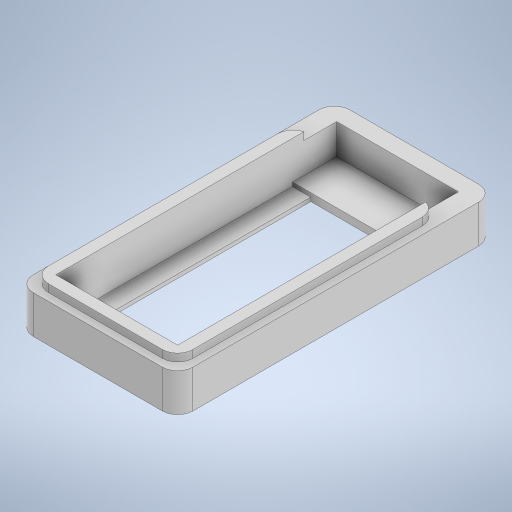
# Autodesk Inventor part: Pieza USB Tester
Saved by Autodesk Inventor 2024 (Build 280153000, 153)
## iProperties
Created: 2023-06-24
Part Number: Pieza USB Tester
Material: Genérico
Document SubType Name: Modeling
Designer: sergi
Density: 1 g/cm^3
Appearance: Valor por defecto
Author: sergi
Autodesk Inventor part; units mm, degrees
ref_plane "YZ Plane" through (0, 0, 0) normal (1, 0, 0) x (0, 1, 0)
ref_plane "XZ Plane" through (0, 0, 0) normal (0, 1, 0) x (-1, 0, 0)
ref_plane "XY Plane" through (0, 0, 0) normal (0, 0, 1) x (1, 0, 0)
sketch "Boceto1" plane through (0, 0, 0) normal (0, 1, 0) x (-1, 0, 0)
  line L0 (-8, -15.55) -> (8, -15.55)
  line L1 (8, -15.55) -> (8, 15.55)
  line L2 (8, 15.55) -> (-8, 15.55)
  line L3 (-8, 15.55) -> (-8, -15.55)
  line L4 (-8, -15.55) -> (8, 15.55) construction
  line L5 (8, -15.55) -> (-8, 15.55) construction
  line L6 (9.5, 17.05) -> (9.5, -17.05)
  line L7 (9.5, -17.05) -> (-9.5, -17.05)
  line L8 (-9.5, -17.05) -> (-9.5, 17.05)
  line L9 (-9.5, 17.05) -> (9.5, 17.05)
  point P0 (0, 0)
  dimension "d0" = 16
  dimension "d1" = 31.1
  dimension "d2" = 1.5
  constraints: 20 end point, 4 parallel, 2 midpoint, 2 perpendicular, 1 horizontal, 3 other
  measures "d0" distance of L2.end L1.end
  measures "d1" distance of L1.end L0.end
  measures "d2" distance between parallel lines of L1 L6
extrude "Extrusión1" add sketch "Boceto1" along normal blind 6
sketch "Boceto2" plane through (0, 0, 0) normal (0, -1, 0) x (1, 0, 0)
  line L0 (9.5, 17.05) -> (9.5, -17.05) projected
  line L1 (-9.5, 17.05) -> (9.5, 17.05) projected
  line L2 (-9.5, -17.05) -> (-9.5, 17.05) projected
  line L3 (9.5, -17.05) -> (-9.5, -17.05) projected
  line L4 (8, -15.55) -> (8, 15.55) projected
  line L5 (-8, -15.55) -> (8, -15.55) projected
  line L6 (-8, 15.55) -> (-8, -15.55) projected
  line L7 (8, 15.55) -> (-8, 15.55) projected
  line L8 (10.5, 18.05) -> (10.5, -18.05)
  line L9 (10.5, -18.05) -> (-10.5, -18.05)
  line L10 (-10.5, -18.05) -> (-10.5, 18.05)
  line L11 (-10.5, 18.05) -> (10.5, 18.05)
  line L12 (10.5, -18.05) -> (-10.5, -18.05)
  line L13 (-10.5, -18.05) -> (-10.5, -24.55)
  line L14 (-10.5, -24.55) -> (10.5, -24.55)
  line L15 (10.5, -24.55) -> (10.5, -18.05)
  point P0 (0, 0)
  dimension "d5" = 2.5
  dimension "d19" = 6.5
  constraints: 16 end point, 2 parallel, 1 horizontal, 1 perpendicular, 3 other
  measures "d5" distance between parallel lines of L4 L8
  measures "d19" distance of L13.end L12.end
extrude "Extrusión2" add sketch "Boceto2" against normal blind 5 contours L0 L3 L2 L1 | L8 L9 L10 L11
sketch "Boceto8" plane through (0, 0, 0) normal (0, -1, 0) x (1, 0, 0)
  line L0 (10.5, 18.05) -> (10.5, -18.05) projected
  line L1 (10.5, -18.05) -> (-10.5, -18.05)
  line L2 (-10.5, -18.05) -> (-10.5, -23.55)
  line L3 (-10.5, -23.55) -> (10.5, -23.55)
  line L4 (10.5, -23.55) -> (10.5, -18.05)
  point P0 (0, 0)
  dimension "d20" = 21
  dimension "d21" = 5.5
  constraints: 8 end point, 2 parallel, 1 horizontal, 1 perpendicular
  measures "d20" distance of L3.end L2.end
  measures "d21" distance of L2.end L1.end
extrude "Extrusión7" add sketch "Boceto8" against normal blind 5
sketch "Boceto9" plane through (0, 6, 0) normal (0, 1, 0) x (1, 0, 0)
  line L0 (9.5, -17.05) -> (9.5, 17.05) projected
  line L1 (9.5, 17.05) -> (-9.5, 17.05) projected
  line L2 (-9.5, 17.05) -> (-9.5, -17.05) projected
  line L3 (-9.5, -17.05) -> (9.5, -17.05) projected
  line L4 (8, 15.55) -> (8, -15.55) projected
  line L5 (8, -15.55) -> (-8, -15.55) projected
  line L6 (-8, -15.55) -> (-8, 15.55) projected
  line L7 (-8, 15.55) -> (8, 15.55) projected
  line L8 (-10.5, 23.55) -> (-10.5, -18.05) projected
  line L9 (-10.5, -18.05) -> (10.5, -18.05) projected
  line L10 (10.5, -18.05) -> (10.5, 23.55) projected
  line L11 (10.5, 23.55) -> (-10.5, 23.55) projected
  line L12 (-9.5, -17.05) -> (9.5, -17.05) projected
  line L13 (-9.5, 17.05) -> (-9.5, -17.05) projected
  line L14 (9.5, 17.05) -> (-9.5, 17.05) projected
  line L15 (9.5, -17.05) -> (9.5, 17.05) projected
  line L16 (-8, 15.55) -> (8, 15.55)
  line L17 (8, 15.55) -> (8, 21.35)
  line L18 (8, 21.35) -> (-8, 21.35)
  line L19 (-8, 21.35) -> (-8, 15.55)
  point P0 (0, 0)
  point P1 (8, 15.55)
  dimension "d24" = 5.8
  constraints: 8 end point, 2 parallel, 1 horizontal, 1 perpendicular
  measures "d24" distance of L17.end L16.end
extrude "Extrusión8" cut sketch "Boceto9" against normal blind 5 contours L17 L7 L19 L1 | L1 L19 L18 L17
fillet "Empalme3" radius 2 4 edges at (-10.5, 2.5, 18.05) (10.5, 2.5, 18.05) (-10.5, 2.5, -23.55) (10.5, 2.5, -23.55)
fillet "Empalme4" radius 2 4 edges at (-9.5, 5.5, -17.05) (-9.5, 5.5, 17.05) (9.5, 5.5, 17.05) (9.5, 5.5, -17.05)
sketch "Boceto10" plane through (0, 0, 0) normal (0, -1, 0) x (1, 0, 0)
  line L0 (8, -15.55) -> (8, 15.55) projected
  line L1 (-8, -15.55) -> (8, -15.55) projected
  line L2 (8, 15.55) -> (5.6, 15.55)
  line L3 (5.6, 15.55) -> (5.6, -15.55)
  line L4 (5.6, -15.55) -> (8, -15.55)
  line L5 (8, -15.55) -> (8, 15.55)
  line L6 (-8, -15.55) -> (-5.6, -15.55)
  line L7 (-5.6, -15.55) -> (-5.6, 15.55)
  line L8 (-5.6, 15.55) -> (-8, 15.55)
  line L9 (-8, 15.55) -> (-8, -15.55)
  point P0 (0, 0)
  dimension "d29" = 2.4
  dimension "d30" = 2.4
  dimension "d31" = 31.1
  constraints: 16 end point, 4 parallel, 2 horizontal, 2 perpendicular, 1 point on line
  measures "d29" distance of L4.end L3.end
  measures "d30" distance of L8.end L7.end
  measures "d31" distance of L7.end L6.end
extrude "Extrusión9" add sketch "Boceto10" against normal blind 0.5
